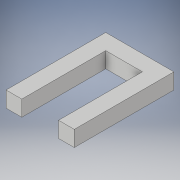
# Autodesk Inventor part: Part3
Saved by Autodesk Inventor 2017 (Build 210142000, 142)
## iProperties
Created: 2017-02-22
Part Number: Part3
Material: Generic
Document SubType Name: Modeling
Designer: John
Density: 1 g/cm^3
Appearance: Default
Author: John
Autodesk Inventor part; units mm, degrees
ref_plane "YZ Plane" through (0, 0, 0) normal (1, 0, 0) x (0, 1, 0)
ref_plane "XZ Plane" through (0, 0, 0) normal (0, 1, 0) x (-1, 0, 0)
ref_plane "XY Plane" through (0, 0, 0) normal (0, 0, 1) x (1, 0, 0)
sketch "Sketch1" plane through (0, 0, 0) normal (0, 1, 0) x (-1, 0, 0)
  line L0 (-13, 0) -> (0, 0)
  line L1 (0, 0) -> (0, 3)
  line L2 (0, 3) -> (-13, 3)
  line L3 (-13, 3) -> (-13, 0)
  line L4 (-13, 3) -> (-10, 3)
  line L5 (-10, 3) -> (-10, 19)
  line L6 (-10, 19) -> (-13, 19)
  line L7 (-13, 19) -> (-13, 3)
  line L8 (0, 3) -> (-3, 3)
  line L9 (-3, 3) -> (-3, 19)
  line L10 (-3, 19) -> (0, 19)
  line L11 (0, 19) -> (0, 3)
  point P0 (0, 0)
  dimension "d0" = 13
  dimension "d1" = 3
  dimension "d2" = 3
  dimension "d3" = 16
  dimension "d4" = 3
  dimension "d5" = 16
  constraints: 24 end point, 6 parallel, 3 horizontal, 3 perpendicular
  measures "d0" distance of L2.end L1.end
  measures "d1" distance of L1.end L0.end
  measures "d2" distance of L6.end L5.end
  measures "d3" distance of L5.end L4.end
  measures "d4" distance of L9.end L10.end
  measures "d5" distance of L8.end L9.end
extrude "Extrusion1" add sketch "Sketch1" along normal blind 3
body "Solid1"
